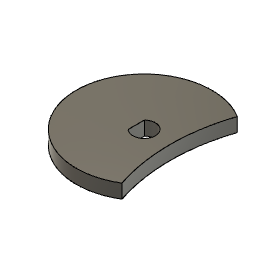
1.DriverWheelTop (Autodesk Fusion 360 design; units mm, degrees)
Autodesk Fusion 360 part; units mm, degrees
sketch "Sketch1" plane through (0, 0, 0) normal (0, 1, 0) x (1, 0, 0)
  arc A0 (10.2337, 16.5989) -> (10.2337, -16.5989) centre (60, 0) ccw
  arc A1 (10.2337, 16.5989) -> (10.2337, -16.5989) centre (0, 0) ccw
  line L0 (-2.25, 2.3452) -> (-2.25, -2.3452)
  arc A2 (-2.25, -2.3452) -> (-2.25, 2.3452) centre (0, 0) ccw
  constraint concentric A1 A2
extrude "Extrude1" add sketch "Sketch1" along normal blind 4
